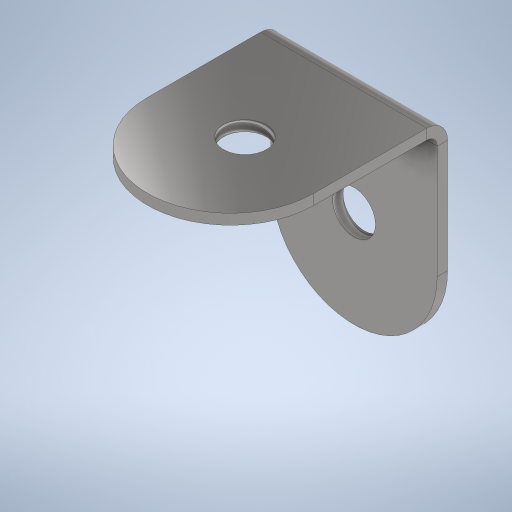
# Autodesk Inventor part: 2309HCMUTE-CDT23_KE-GOC-20X20X16
Saved by Autodesk Inventor 2023 (Build 270158000, 158)
## iProperties
Created: 2023-10-13
Part Number: 2309HCMUTE-CDT23_KE-GOC-20X20X16
Material: Stainless Steel
Document SubType Name: Sheet Metal
Designer: havie
Density: 8 g/cm^3
Sheet Metal Rule: Default_mm
Appearance: Semi-Polished
Author: havie
Autodesk Inventor part; units mm, degrees
ref_plane "YZ Plane" through (0, 0, 0) normal (1, 0, 0) x (0, 1, 0)
ref_plane "XZ Plane" through (0, 0, 0) normal (0, 1, 0) x (-1, 0, 0)
ref_plane "XY Plane" through (0, 0, 0) normal (0, 0, 1) x (1, 0, 0)
sketch "Sketch2" plane through (0, 0, 0.5) normal (0, 0, 1) x (1, 0, 0)
  point P0 (0, 0)
  point P1 (0, 10)
  point P2 (0, -10)
  dimension "d3" = 10
  dimension "d4" = 10
  constraints: 2 vertical alignment
  measures "d3" distance of point (0, 0) point (0, 10)
  measures "d4" distance of point (0, -10) point (0, 0)
sketch "Sketch1" plane through (0, 0, 0) normal (0, 0, 1) x (1, 0, 0)
  line L0 (-8, 20) -> (8, 20)
  line L1 (8, 20) -> (8, -20)
  line L2 (8, -20) -> (-8, -20)
  line L3 (-8, -20) -> (-8, 20)
  line L4 (-8, 20) -> (8, -20) construction
  line L5 (8, 20) -> (-8, -20) construction
  point P0 (0, 0)
  dimension "d0" = 40
  dimension "d1" = 16
  measures "d0" distance of L0.end L1.end
  measures "d1" distance of L0.start L0.end
extrude "Plate1" add sketch "Sketch1" along normal mid plane 1
sketch "Sketch3" plane through (0, 0, 0.5) normal (0, 0, 1) x (1, 0, 0)
  line L0 (-8, -20) -> (-8, 20) projected
  line L1 (-8, 0) -> (8, 0)
  line L2 (8, 20) -> (8, -20) projected
  point P0 (0, 0)
  constraints: 2 end point, 2 midpoint
fold "Fold1" angle 90 bend radius 1 thickness 1 k factor 0.44 line from (-8, 0, 0.5) to (8, 0, 0.5) line at bend centre moving side (0, 1, 0) folds toward (0, 0, 1)
fillet "Corner Round1" radius 8 2 edges at (8, 0.369, 20.369) (-8, 0.369, 20.369)
fillet "Corner Round2" radius 8 2 edges at (-8, -20, 0) (8, -20, 0)
sketch "Sketch4" plane through (0, 0, 0.5) normal (0, 0, 1) x (1, 0, 0)
  line L0 (8, -0.131) -> (-8, -0.131) projected
  line L1 (8, -1.131) -> (8, -0.131) projected
  line L2 (8, -1.131) -> (-8, -1.131) projected
  point P0 (0, 0)
  point P1 (0, -10.631)
  point P2 (8, -0.631)
  point P3 (0, -1.131)
  dimension "d21" = 10
  constraints: 2 midpoint, 1 vertical alignment
  measures "d21" vertical distance of point (8, -0.631) point (0, -10.631)
hole "Hole2" at (0, -10.631, 0.5) direction (0, 0, -1) diameter 4.134 end through all thread size "M5x0.8" class "6H" standard "ISO Metric profile"
sketch "Sketch5" plane through (-8, -0.131, 1.5) normal (0, -1, 0) x (1, 0, 0)
  line L0 (0, 0) -> (0, -1) projected
  line L1 (0, -1) -> (16, -1) projected
  point P0 (8, -1.5)
  point P1 (8, 9.5)
  point P2 (0, -0.5)
  point P3 (8, -1)
  dimension "d29" = 10
  constraints: 2 midpoint, 1 vertical alignment
  measures "d29" vertical distance of point (0, -0.5) point (8, 9.5)
hole "Hole3" at (0, -0.131, 11) direction (0, 1, 0) diameter 4.134 end through all thread size "M5x0.8" class "6H" standard "ISO Metric profile"
equation "\"d2\" = Thickness"
equation "\"d12\" = BendReliefWidth"
equation "\"d13\" = BendReliefDepth"
equation "\"d14\" = MinimumRemnant"
equation "\"d15\" = TransitionRadius"
equation "\"d17\" = BendRadius"
equation "\"BendRadius\" = Thickness"
equation "\"BendReliefWidth\" = Thickness"
equation "\"BendReliefDepth\" = 0.5 * Thickness"
equation "\"CornerReliefSize\" = 4 * Thickness"
equation "\"MinimumRemnant\" = 2 * Thickness"
equation "\"TransitionRadius\" = BendRadius"
equation "\"JacobiRadiusSize\" = BendRadius"
equation "\"GapSize\" = Thickness"
equation "\"Thickness\" = 1"
body "Solid1"
